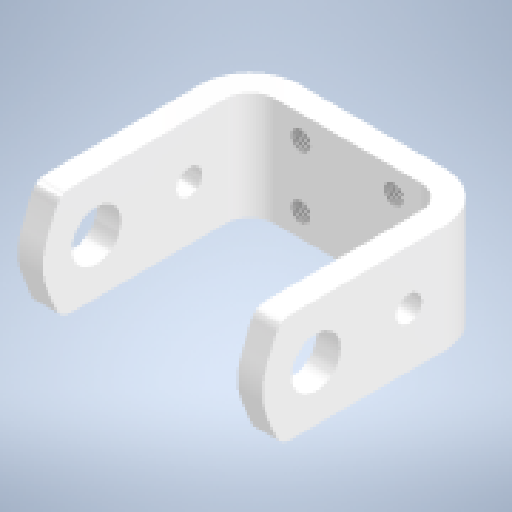
# Autodesk Inventor part: Inductive Probe Mount
Saved by Autodesk Inventor 2024 (Build 280153000, 153)
## iProperties
Created: 2025-01-06
Part Number: Inductive Probe Mount
Material: Aluminum 6061
Document SubType Name: Sheet Metal
Designer: Ishaan
Density: 2.7 g/cm^3
Sheet Metal Rule: SendCutSend_1-8_Alu
Appearance: Aluminum - Flat
Author: Ishaan
Autodesk Inventor part; units mm, degrees
ref_plane "YZ Plane" through (0, 0, 0) normal (1, 0, 0) x (0, 1, 0)
ref_plane "XZ Plane" through (0, 0, 0) normal (0, 1, 0) x (-1, 0, 0)
ref_plane "XY Plane" through (0, 0, 0) normal (0, 0, 1) x (1, 0, 0)
sketch "Sketch1" plane through (0, 0, 0) normal (0, 0, 1) x (1, 0, 0)
  line L0 (12.6, -7) -> (-12.6, -7)
  line L1 (-12.6, -7) -> (-12.6, 7)
  line L2 (-12.6, 7) -> (12.6, 7)
  line L3 (12.6, 7) -> (12.6, -7)
  line L4 (12.6, -7) -> (-12.6, 7) construction
  line L5 (-12.6, -7) -> (12.6, 7) construction
  point P0 (0, 0)
  dimension "d0" = 25.2
  dimension "d1" = 14
  measures "d0" distance of L1.end L2.end
  measures "d1" distance of L0.end L1.end
extrude "Plate1" add sketch "Sketch1" along normal blind 3.175
sketch "Sketch2" plane through (12.6, 7, 3.175) normal (1, 0, 0) x (0, 1, 0)
  line L0 (-14, 0) -> (0, 0)
  line L1 (0, 0) -> (0, 36.825)
  line L2 (0, 36.825) -> (-14, 36.825)
  line L3 (-14, 36.825) -> (-14, 0)
  constraints: 6 end point, 1 horizontal, 1 perpendicular, 1 vertical
edge flange "Flange1" height 40 angle 90 thickness 3.175 bend radius 3.175 thickness toward (1, 0, 0) relief tear relief width 3.175 relief depth 1.5875 corner gap 3.175 corner form 0 edges at (12.6, 0, 3.175) (-12.6, 0, 3.175) wall of the first edge with corners at (12.6, -7, 3.175) (12.6, 7, 3.175) (12.6, 7, 40) (12.6, -7, 40)
bend "Bend1"
corner "Corner1"
sketch "Sketch3" plane through (0, 0, 3.175) normal (0, 0, 1) x (1, 0, 0)
  line L0 (6, -4) -> (-6, -4) construction
  line L1 (-6, -4) -> (-6, 4) construction
  line L2 (-6, 4) -> (6, 4) construction
  line L3 (6, 4) -> (6, -4) construction
  line L4 (6, -4) -> (-6, 4) construction
  line L5 (-6, -4) -> (6, 4) construction
  point P0 (0, 0)
  dimension "d22" = 8
  dimension "d23" = 12
  constraints: 12 end point, 2 coincident, 2 midpoint, 2 parallel, 1 horizontal, 1 perpendicular
  measures "d22" distance of L0.end L1.end
  measures "d23" distance of L1.end L2.end
hole "Hole1" at (-6, 4, 3.175) at (6, -4, 3.175) at (-6, -4, 3.175) at (6, 4, 3.175) direction (0, 0, -1) diameter 2.459 end through all thread size "M3x0.5" class "6H" standard "ANSI Metric M Profile"
sketch "Sketch4" plane through (15.775, -7, 40) normal (1, 0, 0) x (0, 0, -1)
  line L0 (33.65, 0) -> (33.65, 14) projected
  line L1 (0, 14) -> (33.65, 14) projected
  line L2 (0, 0) -> (0, 14) projected
  line L3 (33.65, 0) -> (0, 0) projected
  circle A0 centre (17, 7) radius 7
  line L4 (10.5328, 9.6788) -> (12.3227, 14)
  line L5 (10.5328, 4.3212) -> (12.3227, 0)
  circle A1 centre (29, 7) radius 2.5 construction
  point P0 (40, 7)
  dimension "d24" = 23
  dimension "d25" = 135
  dimension "d36" = 5
  dimension "d37" = 12
  constraints: 4 end point, 4 tangent, 2 centre point, 2 point on circle, 2 point on line, 1 horizontal alignment, 1 vertical alignment
  measures "d24" distance of A0.centre point (40, 7)
  measures "d25" angle of L5 L4
  measures "d36" diameter of A1
  measures "d37" distance of A0.centre A1.centre
extrude "Extrusion1" cut sketch "Sketch4" against normal through all contours L3 L2 L1 L4 A0 L5
sketch "Sketch5" plane through (15.775, -7, 6.35) normal (1, 0, 0) x (0, 0, -1)
  arc A0 (-23.1172, 9.6788) -> (-23.1172, 4.3212) centre (-16.65, 7) ccw projected
  point P0 (6.35, 7)
  constraints: 1 coincident
hole "Hole2" at (15.775, 0, 23) direction (-1, 0, 0) diameter 6.4 end through all
fillet "Fillet1" radius 2 4 edges at (-14.1875, 7, 27.6773) (-14.1875, -7, 27.6773) (14.1875, -7, 27.6773) (14.1875, 7, 27.6773)
hole "Hole3" at (15.775, 0, 11) direction (-1, 0, 0) diameter 3.3 end through all
equation "\"d20\" = Thickness"
equation "\"d2\" = Thickness"
equation "\"d3\" = BendReliefWidth"
equation "\"d4\" = BendReliefDepth"
equation "\"d5\" = MinimumRemnant"
equation "\"d6\" = TransitionRadius"
equation "\"d9\" = BendRadius"
equation "\"d10\" = CornerReliefSize"
equation "\"d11\" = GapSize"
equation "\"d12\" = JacobiRadiusSize"
equation "\"BendReliefWidth\" = Thickness"
equation "\"BendReliefDepth\" = 0.5 * Thickness"
equation "\"CornerReliefSize\" = 4 * Thickness"
equation "\"MinimumRemnant\" = 2 * Thickness"
equation "\"TransitionRadius\" = BendRadius"
equation "\"JacobiRadiusSize\" = BendRadius"
equation "\"GapSize\" = Thickness"
equation "\"Thickness\" = 3.175"
equation "\"BendRadius\" = 3.175"
body "Solid1"
